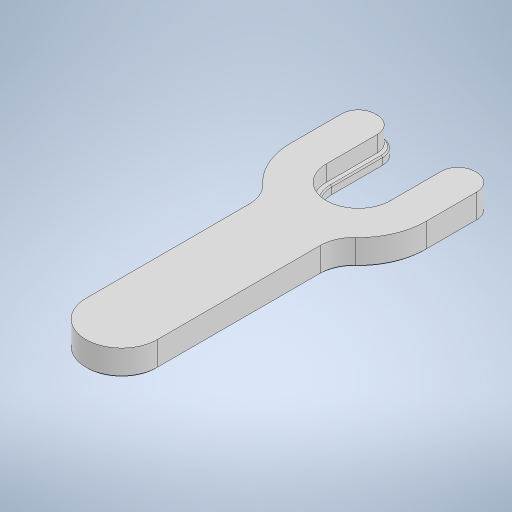
# Autodesk Inventor part: ER11 Collet Removal Tool
Saved by Autodesk Inventor 2023.4 (Build 274418000, 418)
## iProperties
Created: 2024-04-25
Part Number: ER11 Collet Removal Tool
Material: Generic
Document SubType Name: Modeling
Designer: Nathan Cai
Density: 1 g/cm^3
Appearance: Default
Author: Nathan Cai
Autodesk Inventor part; units mm, degrees
ref_plane "YZ Plane" through (0, 0, 0) normal (1, 0, 0) x (0, 1, 0)
ref_plane "XZ Plane" through (0, 0, 0) normal (0, 1, 0) x (-1, 0, 0)
ref_plane "XY Plane" through (0, 0, 0) normal (0, 0, 1) x (1, 0, 0)
sketch "Sketch1" plane through (0, 0, 0) normal (0, 1, 0) x (-1, 0, 0)
  line L0 (0, 0) -> (0, -12.7) construction
  line L1 (-5, 0) -> (-5, -12.7)
  line L2 (5, -12.7) -> (5, 0)
  arc A0 (5, 0) -> (-5, 0) centre (0, 0) ccw
  arc A1 (-5, -12.7) -> (5, -12.7) centre (0, -12.7) ccw construction
  line L3 (0, 0) -> (0, -12.7) construction
  line L4 (-6, 0) -> (-6, -12.7)
  line L5 (6, -12.7) -> (6, 0)
  arc A2 (6, 0) -> (-6, 0) centre (0, 0) ccw
  arc A3 (-6, -12.7) -> (6, -12.7) centre (0, -12.7) ccw construction
  line L6 (0, 0) -> (0, -12.7) construction
  line L7 (-12.7, 0) -> (-12.7, -12.7)
  line L8 (12.7, -12.7) -> (12.7, 0)
  arc A4 (12.7, 0) -> (-12.7, 0) centre (0, 0) ccw
  arc A5 (-12.7, -12.7) -> (12.7, -12.7) centre (0, -12.7) ccw construction
  line L9 (12.7, -12.7) -> (-12.7, -12.7)
  line L10 (0, 12.7) -> (0, 44.45) construction
  line L11 (-6.7, 12.7) -> (-6.7, 44.45)
  line L12 (6.7, 44.45) -> (6.7, 12.7)
  arc A6 (-6.7, 12.7) -> (6.7, 12.7) centre (0, 12.7) ccw
  arc A7 (6.7, 44.45) -> (-6.7, 44.45) centre (0, 44.45) ccw
  point P0 (0, -6.35)
  point P1 (0, -6.35)
  point P2 (0, -6.35)
  point P3 (0, 28.575)
  point P4 (-6.4627, 10.9327)
  point P5 (6.4627, 10.9327)
  dimension "d0" = 12.7
  dimension "d1" = 10
  dimension "d2" = 12
  dimension "d3" = 25.4
  dimension "d4" = 31.75
  constraints: 34 end point, 17 point on circle, 17 tangent, 8 centre point, 6 equal length, 4 midpoint, 2 vertical, 1 horizontal
  measures "d0" distance of L0.start L0.end
  measures "d1" diameter of A1
  measures "d2" diameter of A3
  measures "d3" diameter of A5
  measures "d4" distance of L10.start L10.end
extrude "Extrusion1" add sketch "Sketch1" along normal blind 4.7625 contours L9 L7 A4 A6 A2 L4 | L5 A2 A6 A4 L8 L9 | A6 A4 | A6 L11 A7 L12 A4
extrude "Extrusion2" add sketch "Sketch1" along normal blind 1.75 contours L1 L9 L4 A2 L5 L2 A0
fillet "Fillet1" radius 6.35 2 edges at (-6.4627, 2.3813, 10.9327) (6.4627, 2.3813, 10.9327)
fillet "Fillet2" radius 3.175 4 edges at (-6, 3.2563, -12.7) (6, 3.2563, -12.7) (-5, 0.875, -12.7) (5, 0.875, -12.7)
fillet "Fillet3" radius 3.175 2 edges at (-12.7, 2.3813, -12.7) (12.7, 2.3813, -12.7)
chamfer "Chamfer1" distance 0.25 angle 45 25 edges at (11.7701, 0, -11.7701) (8.85, 0, -12.7) (5.9299, 0, -11.7701) (5, 0, -4.7625) (0, 0, 5) (-5, 0, -4.7625) (-5.9299, 0, -11.7701) (-8.85, 0, -12.7) (-11.7701, 0, -11.7701) (-12.7, 0, -4.7625) (-11.6572, 0, 5.0398) (-7.2214, 0, 11.3581) (-6.7, 0, 29.164) (0, 0, 51.15) (6.7, 0, 29.164) (7.2214, 0, 11.3581) (11.6572, 0, 5.0398) (12.7, 0, -4.7625) (5, 1.75, -4.7625) (0, 1.75, 5) (-5, 1.75, -4.7625) (-5.9299, 1.75, -11.7701) (-8.675, 1.75, -12.7) (5.9299, 1.75, -11.7701) (8.675, 1.75, -12.7)
body "Solid1"
